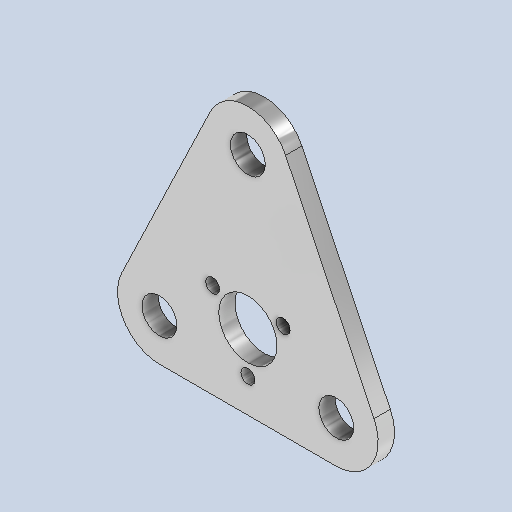
# Autodesk Inventor part: Triangle
Saved by Autodesk Inventor 2023.2 (Build 272271030, 271C)
## iProperties
Created: 2023-03-23
Part Number: Triangle
Material: Nickel-Copper Alloy 400
Document SubType Name: Modeling
Designer: Luis Valente
Density: 8.83 g/cm^3
Appearance: Chrome - Polished
Author: Luis Valente
Autodesk Inventor part; units mm, degrees
ref_plane "YZ Plane" through (0, 0, 0) normal (1, 0, 0) x (0, 1, 0)
ref_plane "XZ Plane" through (0, 0, 0) normal (0, 1, 0) x (-1, 0, 0)
ref_plane "XY Plane" through (0, 0, 0) normal (0, 0, 1) x (1, 0, 0)
sketch "Sketch1" plane through (0, 0, 0) normal (0, 0, 1) x (1, 0, 0)
  line L0 (0, 0) -> (76, 0)
  circle A0 centre (0, 0) radius 7.5
  circle A1 centre (76, 0) radius 7.5
  line L1 (38, 0) -> (38, 115)
  line L2 (38, 115) -> (38, 79)
  circle A2 centre (38, 79) radius 7.5
  arc A3 (54.221, 86.8025) -> (21.779, 86.8025) centre (38, 79) ccw
  arc A4 (-16.221, 7.8025) -> (0, -18) centre (0, 0) ccw
  arc A5 (76, -18) -> (92.221, 7.8025) centre (76, 0) ccw
  line L3 (54.221, 86.8025) -> (92.221, 7.8025)
  line L4 (76, -18) -> (0, -18)
  line L5 (21.779, 86.8025) -> (-16.221, 7.8025)
  line L6 (18, 0) -> (39.1073, 0) construction
  line L7 (38, -18) -> (38, 79)
  point P0 (21.2402, 103.5657)
  point P1 (54.7598, 103.5657)
  dimension "d1" = 76
  dimension "d2" = 15
  dimension "d3" = 15
  dimension "d4" = 115
  dimension "d5" = 36
  dimension "d6" = 15
  dimension "d7" = 36
  dimension "d8" = 36
  dimension "d9" = 36
  dimension "d14" = 97
  constraints: 16 end point, 6 centre point, 6 coincident, 6 point on circle, 6 tangent, 2 horizontal, 2 midpoint, 2 point on line, 1 vertical
  measures "d1" distance of L0.start L0.end
  measures "d2" diameter of A0
  measures "d3" diameter of A1
  measures "d4" distance of L1.start L1.end
  measures "d5" distance of L1.end L2.end
  measures "d6" diameter of A2
  measures "d7" diameter of A3
  measures "d8" diameter of A4
  measures "d9" diameter of A5
  measures "d14" distance of L7.start L7.end
extrude "Extrusion1" add sketch "Sketch1" along normal blind 7 contours L7 L4 A4 L5 A3 L1 A2 | L1 A2 A3 L3 A5 L4 L7
sketch "Sketch3" plane through (0, 0, 7) normal (0, 0, 1) x (1, 0, 0)
  circle A0 centre (76, 0) radius 7.5 projected
  line L0 (76, -7.5) -> (38, -7.5)
  line L1 (0, -18) -> (76, -18) projected
  line L2 (38, -18) -> (38, 14)
  circle A1 centre (38, 14) radius 12.5
  line L3 (38, 14) -> (46.2567, 14) construction
  line L4 (38, 14) -> (59.6506, 26.5)
  line L5 (38, 14) -> (63, 14) construction
  line L6 (38, 14) -> (20.5721, 24.062)
  line L7 (38, 14) -> (58.124, 14) construction
  line L8 (57, -7.5) -> (57, 24.9697)
  line L9 (38, -7.5) -> (0, -7.5)
  circle A2 centre (0, 0) radius 7.5 projected
  line L10 (19, -7.5) -> (19, 24.9697)
  line L11 (19, 24.9697) -> (23.5265, 22.3563)
  line L12 (0, 0) -> (38, 14)
  circle A3 centre (38, 14) radius 17.5
  circle A4 centre (22.8446, 22.75) radius 3
  circle A5 centre (38, -3.5) radius 3
  circle A6 centre (53.1554, 22.75) radius 3
  dimension "d27" = 35
  dimension "d15" = 38
  dimension "d16" = 32
  dimension "d17" = 25
  dimension "d19" = 30
  dimension "d20" = 150
  dimension "d28" = 6
  dimension "d31" = 360
  constraints: 24 end point, 6 horizontal, 4 centre point, 3 midpoint, 3 point on line, 3 vertical, 2 coincident, 2 equal length, 2 vertical alignment, 12 other
  measures "d15" distance of L0.start L0.end
  measures "d16" distance of L2.start L2.end
  measures "d17" diameter of A1
  measures "d19" angle of L5 L4
  measures "d20" angle of L7 L6
  measures "d28" diameter of A4
extrude "Extrusion2" cut sketch "Sketch3" against normal blind 7 contours A5 A3 L2 | L2 A3 A5 | A6 A3 L4 | L4 A3 A6 | A3 A5 L2 | L2 A5 A3 | A3 A6 L4 | L4 A6 A3 | A4 L6 A3 | A3 L6 L11 A4 | A1 L12 L2 | L2 L4 A1 | A1 L6 L12 | A4 L11 L6 A3 | A3 L6 A4 | L4 L6 A1
body "Solid1"
